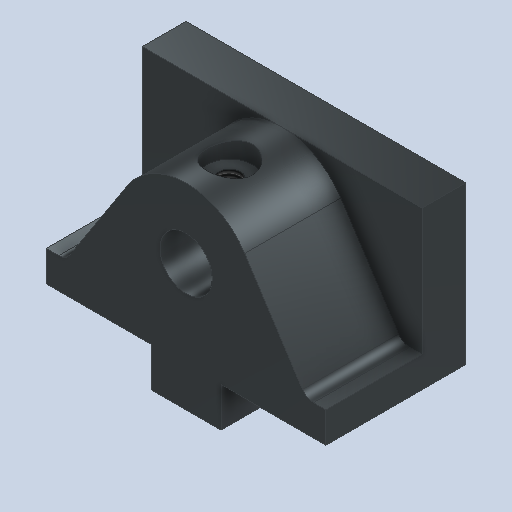
# Autodesk Inventor part: mordente_movel
Saved by Autodesk Inventor 2022.2 (Build 262287010, 287A)
## iProperties
Created: 2022-03-09
Part Number: mordente_movel
Material: Iron, Cast
Document SubType Name: Modeling
Designer: 19710060
Density: 7.15 g/cm^3
Appearance: Iron Gray
Author: 19710060
Autodesk Inventor part; units mm, degrees
ref_plane "YZ Plane" through (0, 0, 0) normal (1, 0, 0) x (0, 1, 0)
ref_plane "XZ Plane" through (0, 0, 0) normal (0, 1, 0) x (-1, 0, 0)
ref_plane "XY Plane" through (0, 0, 0) normal (0, 0, 1) x (1, 0, 0)
sketch "Esboço1" plane through (0, 0, 0) normal (0, 0, 1) x (1, 0, 0)
  line L0 (0, 0) -> (64, 0)
  line L1 (64, 0) -> (64, 45)
  line L2 (64, 45) -> (0, 45)
  line L3 (0, 45) -> (0, 0)
  dimension "d0" = 64
  dimension "d1" = 45
  constraints: 8 end point, 2 parallel, 1 horizontal, 1 perpendicular
  measures "d0" distance of L2.end L1.end
  measures "d1" distance of L1.end L0.end
extrude "Extrusão1" add sketch "Esboço1" against normal blind 32
sketch "Esboço2" plane through (0, 0, 0) normal (0, 0, 1) x (1, 0, 0)
  line L0 (0, 0) -> (0, 9)
  line L1 (0, 0) -> (0, 45) projected
  line L2 (0, 9) -> (24, 9)
  line L3 (24, 9) -> (24, 0)
  line L4 (24, 0) -> (40, 0)
  line L5 (64, 0) -> (0, 0) projected
  line L6 (40, 0) -> (40, 9)
  line L7 (40, 9) -> (64, 9)
  line L8 (64, 45) -> (64, 0) projected
  line L9 (0, 9) -> (0, 16)
  line L10 (64, 9) -> (64, 16)
  circle A0 centre (32, 29) radius 16
  line L11 (45.4187, 37.7142) -> (59.5201, 16)
  line L12 (18.5813, 37.7142) -> (4.4799, 16)
  line L13 (0, 16) -> (4.4799, 16)
  line L14 (59.5201, 16) -> (64, 16)
  line L15 (0, 16) -> (0, 45)
  line L16 (64, 45) -> (0, 45)
  line L17 (64, 45) -> (64, 16)
  point P0 (32, 45)
  dimension "d4" = 9
  dimension "d9" = 7
  constraints: 30 end point, 5 point on line, 3 collinear, 3 perpendicular, 2 point on circle, 2 tangent, 2 vertical, 1 centre point, 1 horizontal
  measures "d4" distance of L0.start L0.end
  measures "d9" distance of L0.end L9.end
extrude "Extrusão2" cut sketch "Esboço2" against normal blind 22 contours L0 L2 L3 L5 | L1 L16 A0 L12 L13 | L6 L7 L8 L5 | L16 L8 L14 L11 A0
sketch "Esboço3" plane through (0, 0, 0) normal (0, 0, 1) x (1, 0, 0)
  line L0 (0, 0) -> (64, 0) projected
  line L1 (32, 0) -> (32, 29)
  point P0 (24, 0)
  point P1 (40, 0)
  dimension "d16" = 29
  constraints: 2 end point, 1 midpoint, 1 vertical
  measures "d16" distance of L1.start L1.end
hole "Furo1" at (32, 29, 0) direction (0, 0, -1) diameter 12 depth 24
fillet "Arredondamento1" radius 3 2 edges at (4.4799, 16, -11) (59.5201, 16, -11)
sketch "Esboço5" plane through (0, 45, 0) normal (0, 1, 0) x (1, 0, 0)
  line L0 (64, 32) -> (0, 32) projected
  line L1 (0, 0) -> (0, 32) projected
  line L2 (0, 32) -> (0, 10)
  line L3 (0, 10) -> (32, 10)
  dimension "d30" = 22
  constraints: 4 end point, 1 horizontal, 1 point on line
  measures "d30" distance of L0.end L2.end
hole "Furo2" at (32, 45, -10) direction (0, -1, 0) diameter 4.917 depth 11 tip angle 118 counterbore diameter 10.5 counterbore depth 4 thread size "M6x1" class "6H" standard "ISO Metric profile"
sketch "Esboço6" plane through (0, 0, -32) normal (0, -1, 0) x (1, 0, 0)
  line L0 (45.4187, 32) -> (18.5813, 32) projected
  line L1 (32, 24) -> (32, 8)
  line L2 (38, 8) -> (26, 8) projected
  point P0 (0, 32)
  dimension "d40" = 16
  constraints: 2 end point, 1 midpoint
  measures "d40" distance of L1.start L1.end
hole "Furo3" at (32, 0, -8) at (32, 0, -24) direction (0, 1, 0) diameter 4.917 depth 12 tip angle 118 thread size "M6x1" class "6H" standard "ISO Metric profile"
sketch "Sketch7" plane through (0, 0, -32) normal (0, -1, 0) x (1, 0, 0)
  line L0 (24, 32) -> (24, 10) projected
  line L1 (24, 10) -> (24, 0)
  line L2 (64, 0) -> (0, 0) projected
  line L3 (0, 0) -> (24, 0)
  line L4 (0, 10) -> (0, 0) projected
  line L5 (0, 0) -> (0, 10)
  line L6 (24, 10) -> (0, 10) projected
  line L7 (0, 10) -> (24, 10)
  line L8 (40, 32) -> (40, 10) projected
  line L9 (40, 10) -> (40, 0)
  line L10 (40, 0) -> (64, 0)
  line L11 (64, 10) -> (64, 0) projected
  line L12 (64, 0) -> (64, 10)
  line L13 (64, 10) -> (40, 10) projected
  line L14 (64, 10) -> (40, 10)
  point P0 (0, 32)
  constraints: 16 end point, 5 collinear, 2 perpendicular, 2 point on line, 1 vertical
extrude "Extrusion3" cut sketch "Sketch7" against normal blind 9
